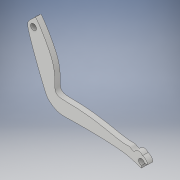
# Autodesk Inventor part: brazo
Saved by Autodesk Inventor 2019 (Build 230136000, 136)
## iProperties
Created: 2019-11-15
Part Number: brazo
Material: Generic
Document SubType Name: Modeling
Designer: Domenico
Density: 1 g/cm^3
Appearance: Default
Author: Domenico
Autodesk Inventor part; units mm, degrees
ref_plane "YZ Plane" through (0, 0, 0) normal (1, 0, 0) x (0, 1, 0)
ref_plane "XZ Plane" through (0, 0, 0) normal (0, 1, 0) x (-1, 0, 0)
ref_plane "XY Plane" through (0, 0, 0) normal (0, 0, 1) x (1, 0, 0)
sketch "Sketch1" plane through (0, 0, 0) normal (0, 0, 1) x (1, 0, 0)
  arc A0 (4.9028, 0.981) -> (0, -5) centre (0, 0) ccw
  line L0 (0, 0) -> (-180, 0) construction
  line L1 (-180, 0) -> (-180, 120) construction
  line L2 (0, 0) -> (-180, 104.9272) construction
  circle A1 centre (-180, 104.9272) radius 5
  line L3 (1.9559, 10.1159) -> (-3.9935, 17.0851) construction
  line L4 (-3.9935, 17.0851) -> (-13.0421, 7.6026) construction
  line L5 (-13.0421, 7.6026) -> (-13.0071, 9.4431) construction
  line L6 (-13.0071, 9.4431) -> (-17.2018, 10.0274) construction
  line L7 (-17.2018, 10.0274) -> (-19.8653, 13.3621) construction
  line L8 (-19.8653, 13.3621) -> (-24.0782, 11.2066) construction
  line L9 (-24.0782, 11.2066) -> (-45.1037, 14.1666) construction
  line L10 (-45.1037, 14.1666) -> (-72.0238, 20.9202) construction
  line L11 (-72.0238, 20.9202) -> (-122.2614, 26.3838) construction
  line L12 (-122.2614, 26.3838) -> (-151.539, 20.9202) construction
  line L13 (-151.539, 20.9202) -> (-137.9781, 56.2422) construction
  line L14 (-137.9781, 56.2422) -> (-155.9397, 90.9018) construction
  line L15 (-155.9397, 90.9018) -> (-176.1289, 122.0426) construction
  line L16 (-176.1289, 122.0426) -> (-177.0156, 120.4623) construction
  spline S0 degree 4 poles (1.9559, 10.1159) (-3.9935, 17.0851) (-13.0421, 7.6026) (-13.0071, 9.4431) (-17.2018, 10.0274) (-19.8653, 13.3621) (-24.0782, 11.2066) (-45.1037, 14.1666) (-72.0238, 20.9202) (-122.2614, 26.3838) (-151.539, 20.9202) (-137.9781, 56.2422) (-155.9397, 90.9018) (-176.1289, 122.0426) (-177.0156, 120.4623) knots 1 1 1 1 1 2 3 4 5 6 7 8 9 10 11 12 12 12 12 12
  line L17 (-177.0156, 120.4623) -> (-188.1506, 111.0524) construction
  line L18 (-188.1506, 111.0524) -> (-190.9564, 106.0524) construction
  line L19 (-190.9564, 106.0524) -> (-189.5534, 98.5339) construction
  line L20 (-189.5534, 98.5339) -> (-180.3933, 70.0684) construction
  line L21 (-180.3933, 70.0684) -> (-157.8506, 13.8118) construction
  line L22 (-157.8506, 13.8118) -> (-156.2384, 13.8118) construction
  line L23 (-156.2384, 13.8118) -> (-141.1398, 0) construction
  line L24 (-141.1398, 0) -> (-122.2614, 1.9224) construction
  line L25 (-122.2614, 1.9224) -> (-95.5749, 1.9224) construction
  line L26 (-95.5749, 1.9224) -> (-73.7351, 1.9224) construction
  line L27 (-73.7351, 1.9224) -> (-22.6011, 0) construction
  line L28 (-22.6011, 0) -> (-13.0663, -5.1287) construction
  line L29 (-13.0663, -5.1287) -> (-0.613, -8.879) construction
  spline S1 degree 4 poles (-177.0156, 120.4623) (-188.1506, 111.0524) (-190.9564, 106.0524) (-189.5534, 98.5339) (-180.3933, 70.0684) (-157.8506, 13.8118) (-156.2384, 13.8118) (-141.1398, 0) (-122.2614, 1.9224) (-95.5749, 1.9224) (-73.7351, 1.9224) (-22.6011, 0) (-13.0663, -5.1287) (-0.613, -8.879) knots 1 1 1 1 1 2 3 4 5 6 7 8 9 10 11 11 11 11 11
  line L30 (0, -8.9002) -> (0, -5)
  line L31 (4.9028, 0.981) -> (10.2564, 0.981)
  arc A2 (10.2564, 0.981) -> (1.9559, 10.1159) centre (0, 0) ccw
  arc A3 (-0.613, -8.879) -> (0, -8.9002) centre (0, 0) ccw
  point P0 (-176.1289, 108.0917)
  dimension "d4" = 10
  dimension "d0" = 10
  dimension "d1" = 180
  dimension "d2" = 120
  dimension "d3" = 208.35
  constraints: 10 end point, 6 point on circle, 6 point on line, 3 centre point, 3 coincident, 2 perpendicular, 2 vertical, 1 horizontal, 1 parallel, 10 other
  measures "d0" diameter of A0
  measures "d1" distance of L0.start L0.end
  measures "d2" distance of L0.end L1.end
  measures "d3" distance of L0.start L2.end
extrude "Extrusion1" add sketch "Sketch1" along normal blind 9
body "Solid1"
